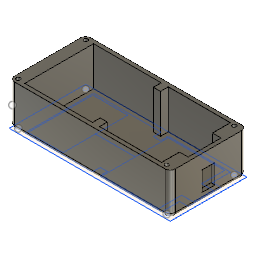
box (Autodesk Fusion 360 design; units mm, degrees)
Autodesk Fusion 360 part; units mm, degrees
sketch "Sketch1" plane through (0, 0, 0) normal (0, 0, 1) x (1, 0, 0)
  line L0 (21.4655, 19.9888) -> (64.9655, 19.9888)
  line L1 (64.9655, 19.9888) -> (64.9655, 2.1388)
  line L2 (64.9655, 2.1388) -> (73.9655, 2.1388)
  line L3 (73.9655, 2.1388) -> (73.9655, -13.1612)
  line L4 (73.9655, -13.1612) -> (64.9655, -13.1612)
  line L5 (64.9655, -13.1612) -> (64.9655, -31.0112)
  line L6 (64.9655, -31.0112) -> (21.4655, -31.0112)
  line L7 (21.4655, -31.0112) -> (21.4655, 19.9888)
  line L8 (-36.1343, 19.4888) -> (-9.1343, 19.4888)
  line L9 (-9.1343, 19.4888) -> (-9.1343, -30.5112)
  line L10 (-9.1343, -30.5112) -> (-36.1343, -30.5112)
  line L11 (-36.1343, -30.5112) -> (-36.1343, 19.4888)
  line L12 (-9.1343, -5.5112) -> (21.4655, -5.5112)
  circle A0 centre (-42.6534, 20.4888) radius 1.5
  circle A1 centre (71.842, 20.4888) radius 1.5
  circle A2 centre (-42.6534, -31.5112) radius 1.5
  circle A3 centre (71.842, -31.5112) radius 1.5
  line L13 (-46.1534, 23.9888) -> (77.9655, 23.9888)
  line L14 (77.9655, 23.9888) -> (77.9655, -35.0112)
  line L15 (77.9655, -35.0112) -> (-46.1534, -35.0112)
  line L16 (-46.1534, -35.0112) -> (-46.1534, 23.9888)
  line L17 (-37.1343, 20.9888) -> (-37.1343, -32.0112)
  line L18 (-37.1343, -32.0112) -> (15.0014, -32.0112)
  line L19 (15.0014, -32.0112) -> (15.0014, -26)
  line L20 (15.0014, -26) -> (20.4655, -26)
  line L21 (20.4655, -26) -> (20.4655, -32.0112)
  line L22 (20.4655, -32.0112) -> (68.342, -32.0112)
  line L23 (68.342, 20.9888) -> (20.4655, 20.9888)
  line L24 (20.4655, 20.9888) -> (20.4655, 14.9776)
  line L25 (20.4655, 14.9776) -> (15.0014, 14.9776)
  line L26 (15.0014, 14.9776) -> (15.0014, 20.9888)
  line L27 (15.0014, 20.9888) -> (-37.1343, 20.9888)
  line L28 (68.342, 20.9888) -> (68.342, 7.1833)
  line L29 (68.342, 7.1833) -> (74.9655, 7.1833)
  line L30 (74.9655, 7.1833) -> (74.9655, -18.2057)
  line L31 (74.9655, -18.2057) -> (68.342, -18.2057)
  line L32 (68.342, -18.2057) -> (68.342, -32.0112)
  dimension "d1" = 52.5
  dimension "d2" = 51
  dimension "d3" = 15.3
  dimension "d4" = 43.5
  dimension "d5" = 50
  dimension "d6" = 27
  dimension "d8" = 3
  dimension "d9" = 3
  dimension "d10" = 3
  dimension "d11" = 3
  dimension "d13" = 1
  dimension "d14" = 1
  dimension "d15" = 1
  dimension "d16" = 1
  dimension "d17" = 3
  dimension "d19" = 3
  dimension "d20" = 3.5
  dimension "d21" = 3.5
  dimension "d22" = 3.5
  dimension "d23" = 3.5
  dimension "d24" = 3.5
  dimension "d26" = 3.5
  dimension "d27" = 3.5
  dimension "d28" = 3.5
  dimension "d31" = 3
  dimension "d35" = 1
  measures "d1" distance of L7
  measures "d2" distance of origin
  measures "d8" diameter of A0
  measures "d9" diameter of A1
  measures "d10" diameter of A2
  measures "d11" diameter of A3
  measures "d13" distance of L6 L22
  measures "d14" distance of L0 L23
  measures "d15" distance of L11 L17
  measures "d16" distance of L3 L30
  measures "d17" distance of L15 L18
  measures "d19" distance of L13 L23
  measures "d24" distance of origin L28
  measures "d27" distance of origin L32
  measures "d31" distance of L14 L30
  measures "d35" distance of L7 L21
extrude "Extrude2" add sketch "Sketch1" along normal blind 33 contours L13 L14 L15 L16 makes body 1
extrude "Extrude1" add sketch "Sketch1" along normal blind 3 separate body contours L0 L1 L2 L3 L4 L5 L6 L7 | L8 L9 L10 L11 | A0 | A1 | A2 | A3 | L13 L14 L15 L16 | L17 L18 L19 L20 L21 L22 L23 L24 L25 L26 L27 L28 L29 L30 L31 L32 makes body 2
combine "Combine1" operation add target body 1 tool bodies 2
fillet "Fillet1" radius 4 7 edges at (77.9655, 23.9888, 16.5) (15.9061, 23.9888, 0) (-46.1534, 23.9888, 16.5) (-46.1534, -5.5112, 0) (-46.1534, -35.0112, 16.5) (15.9061, -35.0112, 0) (77.9655, -35.0112, 16.5) on bodies 1
fillet "Fillet2" radius 4 3 edges at (76.7939, 22.8172, 1.1716) (77.9655, -5.5112, 0) (76.7939, -33.8396, 1.1716) on bodies 1
sketch "Sketch2" plane through (77.9655, 0, 0) normal (1, 0, 0) x (0, 1, 0)
  line L0 (-31.0112, 4) -> (19.9888, 4)
  line L1 (19.9888, 4) -> (19.9888, 33)
  line L2 (19.9888, 33) -> (-31.0112, 33)
  line L3 (-31.0112, 33) -> (-31.0112, 4)
  line L4 (-10.5112, 22) -> (-0.5112, 22)
  line L5 (-0.5112, 22) -> (-0.5112, 7)
  line L6 (-0.5112, 7) -> (-10.5112, 7)
  line L7 (-10.5112, 7) -> (-10.5112, 22)
  line L8 (-5.5112, 7) -> (-5.5112, 4)
  dimension "d38" = 3
  dimension "d39" = 10
  dimension "d40" = 15
  measures "d38" distance of L0 L6
  measures "d39" distance of origin
  measures "d40" distance of L4 L6
extrude "Extrude3" cut sketch "Sketch2" against normal blind 3 contours L4 L5 L6 L7 bodies 1
equation "dia_hole = 3 mm"
equation "d8 = dia_hole"
equation "d9 = dia_hole"
equation "d10 = dia_hole"
equation "d11 = dia_hole"
equation "d20 = dia_hole / 2 + 2 mm"
equation "d21 = dia_hole / 2 + 2 mm"
equation "d22 = dia_hole / 2 + 2 mm"
equation "d23 = dia_hole / 2 + 2 mm"
equation "d24 = dia_hole / 2 + 2 mm"
equation "d26 = dia_hole / 2 + 2 mm"
equation "d27 = dia_hole / 2 + 2 mm"
equation "d28 = dia_hole / 2 + 2 mm"
